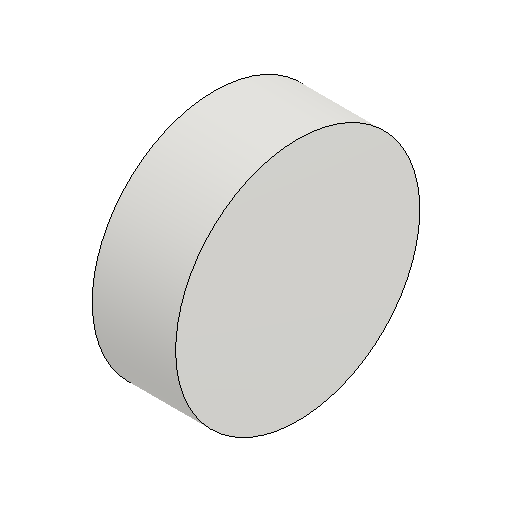
# Autodesk Inventor part: Flat Idler1
Saved by Autodesk Inventor 2025 (Build 290162000, 162)
## iProperties
CustomPartVersion: 1
Created: 2024-07-22
Part Number: Flat Idler1
Material: Steel
Document SubType Name: Modeling
Designer: seene
Density: 1 g/cm^3
Appearance: Steel
Author: seene
Autodesk Inventor part; units mm, degrees
ref_plane "YZ Plane" through (0, 0, 0) normal (1, 0, 0) x (0, 1, 0)
ref_plane "XZ Plane" through (0, 0, 0) normal (0, 1, 0) x (-1, 0, 0)
sketch "Section Profile" plane through (0, 0, 0) normal (0, 0, 1) x (1, 0, 0)
  line L0 (0, 0) -> (7.5225, 0)
  line L1 (7.5225, 0) -> (7.5225, 6.5537)
  line L2 (7.5225, 6.5537) -> (0, 6.5537)
  line L3 (0, 6.5537) -> (0, 0)
  line L4 (0, 0) -> (7.5225, 0)
  line L5 (7.5225, 0) -> (7.5225, 11)
  line L6 (7.5225, 11) -> (0, 11)
  line L7 (0, 11) -> (0, 0)
  point P0 (3.7612, 11)
  dimension "d0" = 7.5225
  dimension "d1" = 7.5225
  dimension "d2" = 3.7612
  dimension "d3" = 13.1074
  dimension "d4" = 22
  constraints: 16 end point, 4 parallel, 2 horizontal, 2 perpendicular, 1 midpoint, 1 point on line
  measures "d0" distance between parallel lines of L5 L7
  measures "d1" distance between parallel lines of L3 L1
  measures "d2" distance from line of point (3.761, 11) L3
  measures "d3" diameter of L2 L0
  measures "d4" diameter of L6 L0
ref_plane "Chain Plane" through (3.7612, 11, 0) normal (1, 0, 0) x (0, 1, 0)
revolve "Shroud" add sketch "Section Profile" angle 360 about axis through (0, 0, 0) along (1, 0, 0) contours L3 L2 L1 L0
revolve "Strand" add sketch "Section Profile" angle 360 about axis through (0, 0, 0) along (1, 0, 0)
pattern_of_one "Strand Pattern"
equation "\"d0\" = da_Bf"
equation "\"d1\" = da_Bs"
equation "\"d3\" = da_Ds"
equation "\"d4\" = da_D"
equation "\"d9\" = da_pt"
equation "\"da_D\" = 22"
equation "\"da_Ds\" = 13.10739"
equation "\"da_Bf\" = 7.52246"
equation "\"da_Bs\" = 7.52246"
equation "\"da_pt\" = 14.3764"
body "Solid1"
